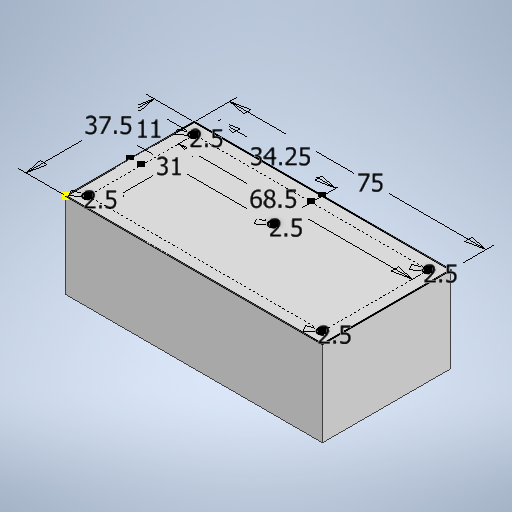
# Autodesk Inventor part: heatsink-CNC
Saved by Autodesk Inventor 2025.2 (Build 292293000, 293)
## iProperties
Created: 2025-05-17
Part Number: heatsink-CNC
Material: Generic
Document SubType Name: Modeling
Designer: user
Density: 1 g/cm^3
Appearance: Default
Author: user
Autodesk Inventor part; units mm, degrees
ref_plane "YZ Plane" through (0, 0, 0) normal (1, 0, 0) x (0, 1, 0)
ref_plane "XZ Plane" through (0, 0, 0) normal (0, 1, 0) x (-1, 0, 0)
ref_plane "XY Plane" through (0, 0, 0) normal (0, 0, 1) x (1, 0, 0)
sketch "Sketch1" plane through (0, 0, 0) normal (0, 1, 0) x (-1, 0, 0)
  line L0 (0, -37.5) -> (-75, -37.5)
  line L1 (-75, -37.5) -> (-75, 0)
  line L2 (-75, 0) -> (0, 0)
  line L3 (0, 0) -> (0, -37.5)
  line L4 (-3.25, -34.25) -> (-71.75, -34.25) construction
  line L5 (-71.75, -34.25) -> (-71.75, -3.25) construction
  line L6 (-71.75, -3.25) -> (-3.25, -3.25) construction
  line L7 (-3.25, -3.25) -> (-3.25, -34.25) construction
  circle A0 centre (-3.25, -34.25) radius 1.25
  circle A1 centre (-37.5, -23.25) radius 1.25
  circle A2 centre (-3.25, -3.25) radius 1.25
  circle A3 centre (-71.75, -3.25) radius 1.25
  circle A4 centre (-71.75, -34.25) radius 1.25
  point P0 (-37.5, -34.25)
  point P1 (-37.5, -37.5)
  point P2 (-3.25, -18.75)
  point P3 (0, -18.75)
  dimension "d0" = 37.5
  dimension "d1" = 75
  dimension "d2" = 31
  dimension "d3" = 68.5
  dimension "d4" = 2.5
  dimension "d6" = 2.5
  dimension "d7" = 2.5
  dimension "d8" = 2.5
  dimension "d9" = 2.5
  dimension "d10" = 34.25
  dimension "d11" = 11
  constraints: 16 end point, 5 centre point, 5 coincident, 4 midpoint, 4 parallel, 2 horizontal, 2 perpendicular, 1 horizontal alignment, 1 vertical alignment
  measures "d0" distance of L2.end L0.start
  measures "d1" distance of L0.start L0.end
  measures "d2" distance of L6.end L4.start
  measures "d3" distance of L4.start L4.end
  measures "d4" diameter of A0
  measures "d6" diameter of A1
  measures "d7" diameter of A2
  measures "d8" diameter of A3
  measures "d9" diameter of A4
  measures "d10" horizontal distance of A1.centre L4.start
  measures "d11" vertical distance of A1.centre L4.start
extrude "Extrusion1" add sketch "Sketch1" against normal blind 25 contours L0 L1 L2 L3 | A0 | A1 | A2 | A3 | A4
extrude "Extrusion2" cut sketch "Sketch1" against normal blind 8 contours A0 | A1 | A2 | A3 | A4
body "Solid1"
